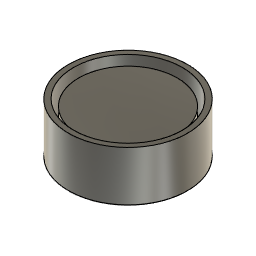
Sorbothane Coasters (Autodesk Fusion 360 design; units mm, degrees)
Autodesk Fusion 360 part; units mm, degrees
sketch "Base " plane through (0, 0, 0) normal (0, 0, 1) x (1, 0, 0)
  circle A0 centre (0, 0) radius 21
  circle A1 centre (0, 0) radius 23
  circle A2 centre (0, 0) radius 6.5
  dimension "d27" = 46
  dimension "d28" = 13
  dimension "d4" = 2
  constraint coincident A0.centre A1.centre
  measures "d27" diameter of A1
  measures "d28" diameter of A2
  measures "d4" distance of A0 A1
extrude "Main Body " add sketch "Base " along normal blind 19.5 contours A1 makes body 1
extrude "Main Body Base" add sketch "Base " along normal blind 2 contours A0 | A2 bodies 1
extrude "Retention Boss" add sketch "Base " along normal blind 2 from surface at 2 contours A2 bodies 1
ref_plane "WorkPlane1" through (0, 0, 14) normal (0, 0, 1) x (1, 0, 0)
sketch "Top" plane through (0, 0, 14) normal (0, 0, 1) x (1, 0, 0)
  circle A0 centre (0, 0) radius 6.5
  circle A1 centre (0, 0) radius 19
  dimension "d21" = 13
  dimension "d22" = 38
  constraint coincident A0.centre A1.centre
  constraint concentric A0 A1
  measures "d21" diameter of A0
  measures "d22" diameter of A1
extrude "Top Extrude" add sketch "Top" along normal blind 3 separate body contours A0 | A1 makes body 2
extrude "Top Retaining Boss" add sketch "Top" against normal blind 2 contours A0 bodies 2
chamfer "Print Surface Fillet" distance 0.3 angle 45 1 edges at (-21.4435, -8.3172, 0) on bodies 1
fillet "Retaining Boss Fillet" radius 1 2 edges at (-6.0601, -2.3505, 4) (-6.0601, 2.3505, 12) on bodies 1 2
sketch "Optional Retaining Ring" plane through (0, 0, 15) normal (0, 0, 1) x (-1, 0, 0)
  circle A0 centre (0, 0) radius 14
  circle A1 centre (0, 0) radius 14
  circle A2 centre (0, 0) radius 13
  dimension "d36" = 26
  constraint concentric A1 A2
  measures "d36" diameter of A2
extrude "Optional glue on ring" [suppressed]
equation "d27 = CupOD"
equation "d28 = RetBossOD"
equation "d4 = WallThickness"
equation "CupOD = SorboRingOD + 8 mm" comment "Cup OD"
equation "SorboRingID = 14 mm" comment "Sorbothane Ring ID"
equation "WallThickness = 2 mm" comment "Wall Thickness"
equation "CupHeight = SorboRingHeight + 7.5 mm" comment "Cup Height"
equation "d9 = CupHeight"
equation "d11 = WallThickness"
equation "SorboRingHeight = 12 mm" comment "Sorbo Ring Height"
equation "SorboRingOD = 38 mm" comment "Sorbo Ring OD"
equation "RetBossHeight = 2 mm" comment "Retaining Boss Height"
equation "d17 = RetBossHeight"
equation "RetBossOD = SorboRingID - 1 mm"
equation "d20 = SorboRingHeight"
equation "d21 = RetBossOD"
equation "d22 = SorboRingOD"
equation "TopHeight = 3 mm" comment "Top Cap Height"
equation "d24 = TopHeight"
equation "d26 = -RetBossHeight"
equation "d32 = RetBossFillet"
equation "RetBossFillet = RetBossHeight / 2" comment "Retaining Boss Fillet"
equation "RubberFootOD = 25 mm" comment "Printer Foot OD"
equation "FootRetRing = RubberFootOD + 1 mm" comment "Retaining Ring OD"
equation "d36 = FootRetRing"
named bodies: "Base", "Top"
